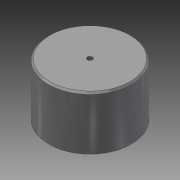
# Autodesk Inventor part: Fixture_Weight
Saved by Autodesk Inventor 2015 (Build 190159000, 159)
## iProperties
Created: 2014-12-16
Part Number: Fixture_Weight
Material: Generic
Document SubType Name: Modeling
Designer: amarschn
Density: 1 g/cm^3
Appearance: Stainless - Brushed
Author: amarschn
Autodesk Inventor part; units mm, degrees
ref_plane "YZ Plane" through (0, 0, 0) normal (1, 0, 0) x (0, 1, 0)
ref_plane "XZ Plane" through (0, 0, 0) normal (0, 1, 0) x (-1, 0, 0)
ref_plane "XY Plane" through (0, 0, 0) normal (0, 0, 1) x (1, 0, 0)
sketch "Sketch2" plane through (0, 0, 0) normal (1, 0, 0) x (0, 1, 0)
  line L0 (0, 0) -> (0, -31.496)
  line L1 (0, -31.496) -> (41.275, -31.496)
  line L2 (41.275, -31.496) -> (41.275, 0)
  line L3 (41.275, 0) -> (0, 0)
  dimension "d0" = 41.275
  dimension "d2" = 31.496
  constraints: 8 end point, 3 perpendicular, 2 point on line, 1 vertical
  measures "d0" distance between parallel lines of L2 L0
  measures "d2" distance of L3.end L0.end
revolve "Revolution1" add sketch "Sketch2" angle 360 about axis through (0, 41.275, 0) along (0, -1, 0)
chamfer "Chamfer1" distance 1.27 angle 45 2 edges at (0, 41.275, 31.496) (0, 0, 31.496)
sketch "Sketch4" plane through (0, 0, 0) normal (0, -1, 0) x (1, 0, 0)
  circle A0 centre (0, 0) radius 3.175 projected
  point P0 (0, 0)
  constraints: 1 coincident
hole "Hole2" at (0, 0, 0) direction (0, 1, 0) diameter 3.302 depth 10.922 tip angle 118 thread size "8-32 UNC" class "2B" standard "ANSI Unified Screw Threads"
sketch "Sketch5" plane through (0, 41.275, 0) normal (0, 1, 0) x (1, 0, 0)
  circle A0 centre (0, 0) radius 1.651 projected
  point P0 (0, 0)
  constraints: 1 coincident
hole "Hole3" at (0, 41.275, 0) direction (0, -1, 0) diameter 3.9624 depth 10.922 tip angle 118 thread size "10-32 UNF" class "2B" standard "ANSI Unified Screw Threads"
body "Solid1"
